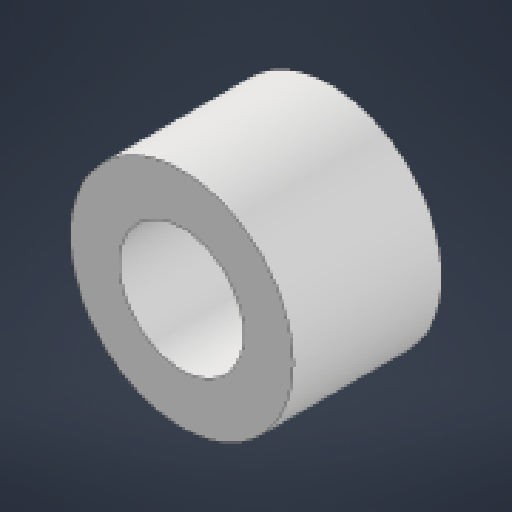
# Autodesk Inventor part: servo_board_spacer
Saved by Autodesk Inventor 2024 (Build 280153000, 153)
## iProperties
Created: 2026-03-28
Part Number: servo_board_spacer
Material: Generic
Document SubType Name: Modeling
Designer: schar
Density: 1 g/cm^3
Appearance: Default
Author: schar
Autodesk Inventor part; units mm, degrees
ref_plane "YZ Plane" through (0, 0, 0) normal (1, 0, 0) x (0, 1, 0)
ref_plane "XZ Plane" through (0, 0, 0) normal (0, 1, 0) x (-1, 0, 0)
ref_plane "XY Plane" through (0, 0, 0) normal (0, 0, 1) x (1, 0, 0)
sketch "Sketch1" plane through (0, 0, 0) normal (0, 0, 1) x (1, 0, 0)
  circle A0 centre (-4.2581, -17.1848) radius 1.25 projected
  circle A1 centre (27.9581, -35.7848) radius 1.25 projected
  circle A2 centre (13.8581, -60.2067) radius 1.25 projected
  circle A3 centre (-18.3581, -41.6067) radius 1.25 projected
  circle A4 centre (-4.2581, -17.1848) radius 2.25
  point P0 (0, 0)
  dimension "d0" = 4.5
  constraints: 1 centre point, 1 coincident
  measures "d0" diameter of A4
extrude "Extrusion1" add sketch "Sketch1" along normal blind 3 contours A4
body "Solid1"
